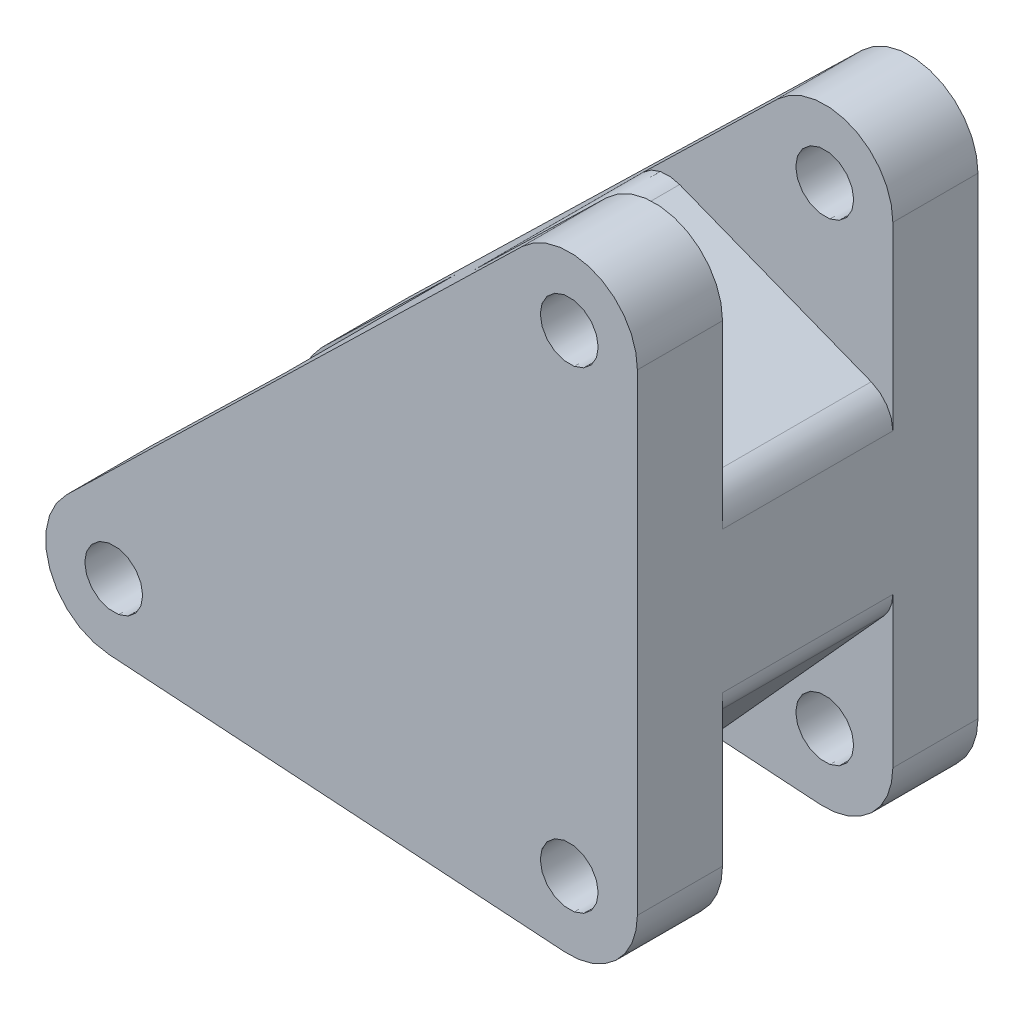
# Autodesk Inventor part: Part2
Saved by Autodesk Inventor 2011 SP2 (Build 150309200, 309)
## iProperties
Created: 2014-05-08
Part Number: Part2
Document SubType Name: Modeling
Designer: Maurice Woods
Density: 1 g/cm^3
ScaleFactor: 1.000 ul
LengthA: 1.000 in
LengthB: 1.092 in
LengthC: 1.034 in
LengthD: 1.055 in
LengthE: 1.468 in
LengthF: 1.037 in
LengthG: 0.966 in
LengthH: 1.729 in
LengthI: 1.289 in
LengthJ: 1.316 in
LengthK: 1.629 in
LengthL: 0.205 in
LengthM: 0.395 in
d0: 1.000 in
d1: 1.316 in
d2: 0.395 in
d3: 0.205 in
d4: 1.092 in
d5: 1.034 in
d7: 1.055 in
d8: 1.468 in
d9: 1.037 in
d10: 0.966 in
d11: 1.729 in
d12: 1.289 in
d13: 1.629 in
Author: Maurice Woods
Autodesk Inventor part; units mm, degrees
ref_plane "YZ Plane" through (0, 0, 0) normal (1, 0, 0) x (0, 1, 0)
ref_plane "XZ Plane" through (0, 0, 0) normal (0, 1, 0) x (-1, 0, 0)
ref_plane "XY Plane" through (0, 0, 0) normal (0, 0, 1) x (1, 0, 0)
sketch "Sketch1" plane through (0, 0, 0) normal (0, 0, 1) x (1, 0, 0)
  line L0 (0, 0) -> (-26.7469, 1.7445) construction
  line L1 (-26.7469, 1.7445) -> (0, 27.7395) construction
  line L2 (0, 27.7395) -> (0, 0) construction
  line L3 (-0.2603, -3.9915) -> (-27.0072, -2.247)
  line L4 (-29.5347, 4.6129) -> (-2.7878, 30.6079)
  line L5 (4, 27.7395) -> (4, 0)
  arc A0 (4, 27.7395) -> (-2.7878, 30.6079) centre (0, 27.7395) ccw
  arc A1 (-29.5347, 4.6129) -> (-27.0072, -2.247) centre (-26.7469, 1.7445) ccw
  arc A2 (-0.2603, -3.9915) -> (4, 0) centre (0, 0) ccw
  dimension "d6" = 37.2979
  dimension "d14" = 27.7395
  dimension "d15" = 26.8037
  dimension "d18" = 4
  constraints: 12 end point, 6 point on circle, 6 tangent, 3 centre point, 2 coincident, 2 equal radius, 1 vertical, 2 other
  measures "d6" distance of L0.end L1.end
  measures "d14" distance of L1.end L0.start
  measures "d15" distance of L0.start L0.end
  measures "d18" radius of A0
extrude "Extrusion1" add sketch "Sketch1" along normal mid plane 20
sketch "Sketch2" plane through (0, 0, 0) normal (0, 0, 1) x (1, 0, 0)
  arc A0 (4, 27.7395) -> (-2.7878, 30.6079) centre (0, 27.7395) ccw
  line L0 (-29.5347, 4.6129) -> (-22.4577, 11.491)
  arc A1 (-29.5347, 4.6129) -> (-27.0072, -2.247) centre (-26.7469, 1.7445) ccw
  line L1 (-0.2603, -3.9915) -> (-6.5178, -3.5834)
  arc A2 (-0.2603, -3.9915) -> (4, 0) centre (0, 0) ccw
  line L2 (4, 27.7395) -> (4, 18.501)
  line L3 (-22.4577, 11.491) -> (-19.1785, -2.7576)
  line L4 (-22.4577, 11.491) -> (-9.7194, 23.8712) construction
  line L5 (-19.1785, -2.7576) -> (-27.0072, -2.247)
  line L6 (-9.7194, 23.8712) -> (4, 18.501)
  line L7 (4, 8.052) -> (-6.5178, -3.5834)
  line L8 (4, 18.501) -> (4, 8.052) construction
  line L9 (4, 8.052) -> (4, 0)
  line L10 (-6.5178, -3.5834) -> (-19.1785, -2.7576) construction
  line L11 (-9.7194, 23.8712) -> (-2.7878, 30.6079)
  arc A3 (-0.2603, -3.9915) -> (4, 0) centre (0, 0) ccw projected
  point P0 (0, 0)
  constraints: 24 end point, 6 centre point, 6 point on circle, 5 collinear, 3 tangent, 1 point on line, 1 vertical, 6 other
extrude "Extrusion2" cut sketch "Sketch2" along normal mid plane 10
sketch "Sketch3" plane through (0, 0, 10) normal (0, 0, 1) x (1, 0, 0)
  arc A0 (4, 27.7395) -> (-2.7878, 30.6079) centre (0, 27.7395) ccw construction
  arc A1 (-29.5347, 4.6129) -> (-27.0072, -2.247) centre (-26.7469, 1.7445) ccw construction
  arc A2 (-0.2603, -3.9915) -> (4, 0) centre (0, 0) ccw construction
hole "Hole1" at (-26.7469, 1.7445, 10) at (0, 0, 10) at (0, 27.7395, 10) direction (0, 0, -1) diameter 3.4 end through all clearance for "Socket Head Cap Screw" size "M3" standard "Ansi Metric M Profile"
fillet "Fillet1" radius 2 6 edges at (-19.1785, -2.7576, 0) (-6.5178, -3.5834, 0) (-22.4577, 11.491, 0) (-9.7194, 23.8712, 0) (4, 18.501, 0) (4, 8.052, 0)
equation "\"d6\" = LengthE"
equation "\"d14\" = LengthB"
equation "\"d15\" = LengthD"
equation "\"ScaleFactor\" = 1"
equation "\"LengthA\" = 25.4 * ScaleFactor"
equation "\"LengthB\" = 27.7395 * ScaleFactor"
equation "\"LengthC\" = 26.269 * ScaleFactor"
equation "\"LengthD\" = 26.8037 * ScaleFactor"
equation "\"LengthE\" = 37.2979 * ScaleFactor"
equation "\"LengthF\" = 26.3358 * ScaleFactor"
equation "\"LengthG\" = 24.531 * ScaleFactor"
equation "\"LengthH\" = 43.9153 * ScaleFactor"
equation "\"LengthI\" = 32.7525 * ScaleFactor"
equation "\"LengthJ\" = 33.421 * ScaleFactor"
equation "\"LengthK\" = 41.3753 * ScaleFactor"
equation "\"LengthL\" = 5.21368 * ScaleFactor"
equation "\"LengthM\" = 10.0263 * ScaleFactor"
equation "\"d0\" = LengthA"
equation "\"d1\" = LengthJ"
equation "\"d2\" = LengthM"
equation "\"d3\" = LengthL"
equation "\"d4\" = LengthB"
equation "\"d5\" = LengthC"
equation "\"d7\" = LengthD"
equation "\"d8\" = LengthE"
equation "\"d9\" = LengthF"
equation "\"d10\" = LengthG"
equation "\"d11\" = LengthH"
equation "\"d12\" = LengthI"
equation "\"d13\" = LengthK"
body "Solid1"
